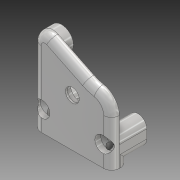
# Autodesk Inventor part: phalanx_3_housing_L
Saved by Autodesk Inventor 2017 SP1 (Build 210196100, 196)
## iProperties
Created: 2017-06-05
Part Number: phalanx_3_housing_L
Material: Generic
Document SubType Name: Modeling
Designer: Tomasz
Density: 1 g/cm^3
Appearance: Aluminum - Polished
Author: Tomasz
Autodesk Inventor part; units mm, degrees
ref_plane "YZ Plane" through (0, 0, 0) normal (1, 0, 0) x (0, 1, 0)
ref_plane "XZ Plane" through (0, 0, 0) normal (0, 1, 0) x (-1, 0, 0)
ref_plane "XY Plane" through (0, 0, 0) normal (0, 0, 1) x (1, 0, 0)
sketch "Sketch1" plane through (0, 0, 0) normal (0, 1, 0) x (-1, 0, 0)
  line L0 (-5, 4.5) -> (5, 4.5)
  line L1 (10, -0.5) -> (10, -12.2)
  line L2 (10, -12.2) -> (-10, -12.2)
  line L3 (-10, -12.2) -> (-10, -0.5)
  line L4 (0, 0) -> (0, -71.875) construction
  arc A0 (10, -0.5) -> (5, 4.5) centre (5, -0.5) ccw
  arc A1 (-5, 4.5) -> (-10, -0.5) centre (-5, -0.5) ccw
  point P0 (-10, 4.5)
  point P1 (10, 4.5)
  dimension "d0" = 20
  dimension "d1" = 12.2
  dimension "d2" = 4.5
  dimension "d32" = 5
  dimension "d33" = 5
  constraints: 10 end point, 4 point on circle, 4 point on line, 4 tangent, 2 centre point, 2 parallel, 1 horizontal, 1 perpendicular, 1 vertical, 1 other
  measures "d0" distance between parallel lines of L3 L1
  measures "d1" distance from line of L2 L4.start
  measures "d2" distance from line of L4.start L0
  measures "d32" radius of A0
  measures "d33" radius of A1
extrude "Extrusion1" add sketch "Sketch1" along normal blind 2
sketch "Sketch2" plane through (0, 2, 0) normal (0, 1, 0) x (1, 0, 0)
  circle A0 centre (0, 0) radius 2.5
  dimension "d6" = 5
  constraints: 1 centre point, 1 coincident
  measures "d6" diameter of A0
extrude "Extrusion2" cut sketch "Sketch2" against normal blind 1.5
hole "Hole1" at (0, 0.5, 0) direction (0, -1, 0) diameter 3.5 end through all
sketch "Sketch4" plane through (0, 0, 0) normal (0, -1, 0) x (1, 0, 0)
  arc A0 (-5.687944, 9.697871) -> (-10, 7) centre (-7, 7) ccw
  line L0 (10, -0.5) -> (10, -12.2)
  arc A1 (10, -0.5) -> (5, 4.5) centre (5, -0.5) ccw
  line L1 (-5, 4.5) -> (5, 4.5)
  arc A2 (-5, 4.5) -> (-10, -0.5) centre (-5, -0.5) ccw
  line L2 (-10, -12.2) -> (-10, -0.5)
  line L3 (-10, -12.2) -> (-10, -0.5)
  line L4 (-10, 7) -> (-10, -0.5)
  line L5 (-5, 4.5) -> (5, 4.5)
  line L6 (-5.687944, 9.697871) -> (5, 4.5)
  line L7 (10, -12.2) -> (-10, -12.2)
  point P0 (0, 0)
  dimension "d34" = 7
  dimension "d35" = 7
  constraints: 4 end point, 3 point on circle, 3 tangent, 1 centre point, 1 vertical
  measures "d34" horizontal distance of A0.centre point (0, 0)
  measures "d35" horizontal distance of point (0, 0) A0.centre
extrude "Extrusion4" add sketch "Sketch4" against normal up to surface (2 mm away) contours L6 L1 A2 L4 A0
fillet "Fillet1" radius 10 1 edges at (5, 1, 4.5)
sketch "Sketch5" plane through (10, 2, -0.5) normal (0, 1, 0) x (1, 0, 0)
  arc A0 (-15.687944, -10.197871) -> (-20, -7.5) centre (-17, -7.5) ccw
  circle A1 centre (-17, -7.5) radius 3
  point P0 (-10, -0.5)
  constraints: 1 centre point, 1 coincident, 1 concentric
extrude "Extrusion5" add sketch "Sketch5" along normal blind 2.25
hole "Hole3" at (-7, 4.25, 7) direction (0, -1, 0) diameter 1.5 depth 3 tip angle 118
sketch "Sketch6" plane through (0, 2, 0) normal (0, 1, 0) x (1, 0, 0)
  arc A0 (-5.687944, -9.697871) -> (-10, -7) centre (-7, -7) ccw
  line L0 (3.500718, -5.229146) -> (-5.687944, -9.697871)
  arc A1 (5.95808, -4.40735) -> (3.500718, -5.229146) centre (7.874239, -14.22205) ccw
  arc A2 (5.95808, -4.40735) -> (10, 0.5) centre (5, 0.5) ccw
  line L1 (10, 0.5) -> (10, 12.2)
  line L2 (10, 12.2) -> (-10, 12.2)
  line L3 (-10, 12.2) -> (-10, -7)
  circle A3 centre (0, 0) radius 2.5
  line L4 (-10, 12.2) -> (10, 12.2)
  line L5 (10, 12.2) -> (10, 9.2)
  line L6 (10, 9.2) -> (-10, 9.2)
  line L7 (-10, 9.2) -> (-10, 12.2)
  dimension "d65" = 3
  constraints: 8 end point, 2 parallel, 1 horizontal, 1 perpendicular, 1 point on line
  measures "d65" distance between parallel lines of L2 L6
extrude "Extrusion6" add sketch "Sketch6" along normal blind 2.25 contours L3 L2 L1 L6
sketch "Sketch7" plane through (0, 0, 0) normal (0, -1, 0) x (1, 0, 0)
  circle A0 centre (0, 0) radius 1.75
  line L0 (-10, -12.2) -> (-10, 7)
  line L1 (10, -12.2) -> (-10, -12.2)
  line L2 (10, -0.5) -> (10, -12.2)
  arc A1 (10, -0.5) -> (5.95808, 4.40735) centre (5, -0.5) ccw
  arc A2 (3.500718, 5.229146) -> (5.95808, 4.40735) centre (7.874239, 14.22205) ccw
  line L3 (3.500718, 5.229146) -> (-5.687944, 9.697871)
  arc A3 (-5.687944, 9.697871) -> (-10, 7) centre (-7, 7) ccw
  line L4 (0, -12.2) -> (0, -3.411922) construction
  line L5 (-16, -6.95) -> (18, -6.95) construction
  arc A4 (10, -6.95) -> (5.5, -6.95) centre (7.75, -6.95) ccw
  arc A5 (-5.5, -6.95) -> (-10, -6.95) centre (-7.75, -6.95) ccw
  line L6 (-10, -12.2) -> (-10, 7)
  line L7 (10, -0.5) -> (10, -12.2)
  line L8 (-10, -9.2) -> (10, -9.2)
  line L9 (5.5, -6.95) -> (5.5, -9.2)
  line L10 (10, -9.2) -> (-10, -9.2)
  line L11 (-5.5, -6.95) -> (-5.5, -9.2)
  arc A6 (5.5, -9.2) -> (10, -9.2) centre (7.75, -9.2) ccw
  line L12 (10, -6.95) -> (10, -9.2)
  line L13 (-10, -9.2) -> (-10, 7)
  line L14 (-10, -6.95) -> (-10, -9.2)
  arc A7 (-10, -9.2) -> (-5.5, -9.2) centre (-7.75, -9.2) ccw
  dimension "d68" = 5.25
  dimension "d69" = 2.25
  constraints: 13 point on line, 12 end point, 9 point on circle, 6 tangent, 4 centre point, 2 coincident, 2 vertical, 1 collinear, 1 horizontal, 1 midpoint, 1 perpendicular, 1 symmetric about line
  measures "d68" distance between parallel lines of L5 L1
  measures "d69" distance from line of point (-7.75, -6.95) L0
sketch "Sketch9" plane through (-7, 4.25, 7) normal (0, 1, 0) x (1, 0, 0)
  circle A0 centre (0, 0) radius 0.75 projected
  circle A1 centre (0, 0) radius 3 projected
  circle A2 centre (0, 0) radius 0.75 projected
  circle A3 centre (0, 0) radius 1.25
  point P0 (7, 7)
  dimension "d88" = 2.5
  constraints: 1 centre point, 1 coincident
  measures "d88" diameter of A3
extrude "Extrusion7" add sketch "Sketch9" along normal blind 0.3 contours A3
extrude "Extrusion8" add sketch "Sketch7" against normal blind 9 contours L0 A5 L11 L8 | L8 A7 | L8 L9 A4 L2 | A6 L8
fillet "Fillet2" radius 2.1 2 edges at (-5.5, 3.125, -9.2) (5.5, 3.125, -9.2)
sketch "Sketch8" plane through (10, 0, -12.2) normal (0, 0, -1) x (-1, 0, 0)
  line L0 (0, 0) -> (20, 0) projected
  line L1 (20, 0) -> (20, 4.25) projected
  line L2 (0, 4.25) -> (20, 4.25) projected
  line L3 (0, 0) -> (0, 4.25) projected
  line L4 (10, 0) -> (10, 4.25) construction
  line L5 (20, 2.2) -> (0, 2.2) construction
  line L6 (0, 0) -> (0, 4.25) projected
  point P0 (17.5, 2.2)
  point P1 (2.5, 2.2)
  dimension "d77" = 2.2
  dimension "d78" = 15
  constraints: 4 end point, 4 point on line, 1 midpoint, 1 perpendicular, 1 symmetric about line
  measures "d77" distance between parallel lines of L0 L5
  measures "d78" distance of point (2.5, 2.2) point (17.5, 2.2)
hole "Hole6" at (-7.5, 2.2, -12.2) at (7.5, 2.2, -12.2) direction (0, 0, 1) diameter 1.6 depth 4 tip angle 118
sketch "Sketch11" plane through (0, 0, 0) normal (0, -1, 0) x (1, 0, 0)
  arc A0 (10, -6.95) -> (5.5, -6.95) centre (7.75, -6.95) ccw projected
  arc A1 (-5.5, -6.95) -> (-10, -6.95) centre (-7.75, -6.95) ccw projected
  point P0 (0, 0)
  constraints: 2 coincident
hole "Hole9" at (-7.75, 0, -6.95) at (7.75, 0, -6.95) direction (0, 1, 0) diameter 4 depth 1.5
sketch "Sketch12" plane through (-7.75, 1.5, -6.95) normal (0, -1, 0) x (0.9918446, 0, 0.1274528)
  arc A0 (0.390483, -1.96151) -> (-0.390483, -1.96151) centre (0, 0) ccw
  arc A1 (15.255466, -3.972027) -> (14.499873, -3.774578) centre (15.373592, -1.975518) ccw
  line L0 (14.582175, -3.134099) -> (14.499873, -3.774578)
  line L1 (15.255466, -3.972027) -> (15.350454, -3.232823)
  line L2 (-0.295495, -1.222307) -> (-0.390483, -1.96151)
  line L3 (0.390483, -1.96151) -> (0.472785, -1.321031)
  point P0 (8.572593, 5.905561)
  constraints: 2 other
hole "Hole10" at (-7.75, 1.5, -6.95) at (7.75, 1.5, -6.95) direction (0, 1, 0) diameter 2.4 end through all countersink diameter 4 countersink angle 90
fillet "Fillet3" radius 2 10 edges at (-8.5912, 0, 9.5432) (-1.0936, 0, 7.4635) (4.7027, 0, 4.7383) (8.8594, 0, 2.6788) (10, 0, -10.7) (10, 0, -8.075) (10, 0, -3.725) (-10, 0, 0.025) (-10, 0, -8.075) (-10, 0, -10.7)
fillet "Fillet4" radius 2 2 edges at (-10, 4.25, -10.7) (10, 4.25, -10.7)
equation "\"d66\" = encoder_mount_height"
equation "\"d68\" = dist_screw_mount_point_1"
equation "\"d69\" = dist_screw_mount_point_2"
equation "\"d77\" = fingertip_mounting_dist_from_edge"
equation "\"d78\" = fingertip_mount_spacing"
equation "\"shaft_to_encoder_mount_points\" = 10.7"
equation "\"dist_screw_mount_point_1\" = 5.25"
equation "\"dist_screw_mount_point_2\" = 2.25"
equation "\"fingertip_mount_spacing\" = 15"
equation "\"encoder_mount_height\" = 2.25"
equation "\"fingertip_mounting_dist_from_edge\" = 2.2"
body "Solid1"
